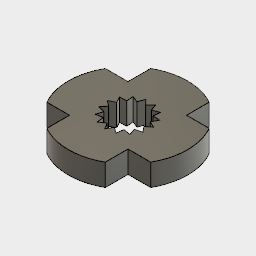
servo_horn_through_hole (Autodesk Fusion 360 design; units mm, degrees)
Autodesk Fusion 360 part; units mm, degrees
sketch "スケッチ1" plane through (0, 0, 0) normal (0, 1, 0) x (1, 0, 0)
  circle A0 centre (0, 0) radius 5.4
  line L0 (2.65, -2.65) -> (-2.65, -2.65)
  line L1 (-2.65, -2.65) -> (-2.65, 2.65)
  line L2 (-2.65, 2.65) -> (2.65, 2.65)
  line L3 (2.65, 2.65) -> (2.65, -2.65)
  line L4 (2.65, -2.65) -> (-2.65, 2.65) construction
  line L5 (-2.65, -2.65) -> (2.65, 2.65) construction
  line L6 (2.65, 2.65) -> (4.7051, 2.65)
  line L7 (2.65, 2.65) -> (2.65, 4.7051)
  line L8 (-2.65, 2.65) -> (-4.7051, 2.65)
  line L9 (-2.65, 2.65) -> (-2.65, 4.7051)
  line L10 (-2.65, -2.65) -> (-4.7051, -2.65)
  line L11 (-2.65, -2.65) -> (-2.65, -4.7051)
  line L12 (2.65, -2.65) -> (2.65, -4.7051)
  line L13 (2.65, -2.65) -> (4.7051, -2.65)
  dimension "d1" = 10.8
  dimension "d4" = 5.3
  dimension "d5" = 5.3
  constraint perpendicular L0 L1
  constraint parallel L0 L2
  constraint parallel L1 L3
  constraint horizontal L0
  constraint coincident L4
  constraint coincident L5
  constraint coincident A0
  constraint perpendicular L3 L6
  constraint perpendicular L6 L7
  constraint perpendicular L7 L8
  constraint perpendicular L8 L9
  constraint perpendicular L9 L10
  constraint perpendicular L10 L11
  constraint perpendicular L0 L12
  constraint perpendicular L12 L13
  measures "d1" diameter of A0
sketch "スケッチ2" plane through (0, 0, 0) normal (0, 1, 0) x (1, 0, 0)
  line L0 (0, -2.102) -> (0.855, -1.9203)
  line L1 (0.855, -1.9203) -> (1.5621, -1.4065)
  line L2 (1.5621, -1.4065) -> (1.9991, -0.6496)
  line L3 (1.9991, -0.6496) -> (2.0905, 0.2197)
  line L4 (2.0905, 0.2197) -> (1.8204, 1.051)
  line L5 (1.8204, 1.051) -> (1.2355, 1.7006)
  line L6 (1.2355, 1.7006) -> (0.437, 2.0561)
  line L7 (0.437, 2.0561) -> (-0.437, 2.0561)
  line L8 (-0.437, 2.0561) -> (-1.2355, 1.7006)
  line L9 (-1.2355, 1.7006) -> (-1.8204, 1.051)
  line L10 (-1.8204, 1.051) -> (-2.0905, 0.2197)
  line L11 (-2.0905, 0.2197) -> (-1.9991, -0.6496)
  line L12 (-1.9991, -0.6496) -> (-1.5621, -1.4065)
  line L13 (-1.5621, -1.4065) -> (-0.855, -1.9203)
  line L14 (-0.855, -1.9203) -> (0, -2.102)
  line L15 (0, 1.6) -> (-0.6508, 1.4617)
  line L16 (-0.6508, 1.4617) -> (-1.189, 1.0706)
  line L17 (-1.189, 1.0706) -> (-1.5217, 0.4944)
  line L18 (-1.5217, 0.4944) -> (-1.5912, -0.1672)
  line L19 (-1.5912, -0.1672) -> (-1.3856, -0.8)
  line L20 (-1.3856, -0.8) -> (-0.9405, -1.2944)
  line L21 (-0.9405, -1.2944) -> (-0.3327, -1.565)
  line L22 (-0.3327, -1.565) -> (0.3327, -1.565)
  line L23 (0.3327, -1.565) -> (0.9405, -1.2944)
  line L24 (0.9405, -1.2944) -> (1.3856, -0.8)
  line L25 (1.3856, -0.8) -> (1.5912, -0.1672)
  line L26 (1.5912, -0.1672) -> (1.5217, 0.4944)
  line L27 (1.5217, 0.4944) -> (1.189, 1.0706)
  line L28 (1.189, 1.0706) -> (0.6508, 1.4617)
  line L29 (0.6508, 1.4617) -> (0, 1.6)
  line L30 (0, -2.102) -> (0.3327, -1.565)
  line L31 (0.3327, -1.565) -> (0.855, -1.9203)
  line L32 (0.855, -1.9203) -> (0.9405, -1.2944)
  line L33 (0.9405, -1.2944) -> (1.5621, -1.4065)
  line L34 (1.5621, -1.4065) -> (1.3856, -0.8)
  line L35 (1.3856, -0.8) -> (1.9991, -0.6496)
  line L36 (1.5912, -0.1672) -> (1.9991, -0.6496)
  line L37 (1.5912, -0.1672) -> (2.0905, 0.2197)
  line L38 (2.0905, 0.2197) -> (1.5217, 0.4944)
  line L39 (1.8204, 1.051) -> (1.5217, 0.4944)
  line L40 (1.8204, 1.051) -> (1.189, 1.0706)
  line L41 (1.2355, 1.7006) -> (1.189, 1.0706)
  line L42 (1.2355, 1.7006) -> (0.6508, 1.4617)
  line L43 (0.437, 2.0561) -> (0.6508, 1.4617)
  line L44 (0.437, 2.0561) -> (0, 1.6)
  line L45 (0, 1.6) -> (-0.437, 2.0561)
  line L46 (-0.437, 2.0561) -> (-0.6508, 1.4617)
  line L47 (-1.2355, 1.7006) -> (-0.6508, 1.4617)
  line L48 (-1.2355, 1.7006) -> (-1.189, 1.0706)
  line L49 (-1.189, 1.0706) -> (-1.8204, 1.051)
  line L50 (-1.8204, 1.051) -> (-1.5217, 0.4944)
  line L51 (-1.5217, 0.4944) -> (-2.0905, 0.2197)
  line L52 (-2.0905, 0.2197) -> (-1.5912, -0.1672)
  line L53 (-1.5912, -0.1672) -> (-1.9991, -0.6496)
  line L54 (-1.9991, -0.6496) -> (-1.3856, -0.8)
  line L55 (-1.3856, -0.8) -> (-1.5621, -1.4065)
  line L56 (-1.5621, -1.4065) -> (-0.9405, -1.2944)
  line L57 (-0.855, -1.9203) -> (-0.9405, -1.2944)
  line L58 (-0.855, -1.9203) -> (-0.3327, -1.565)
  line L59 (-0.3327, -1.565) -> (0, -2.102)
extrude "押し出し1" add sketch "スケッチ1" along normal blind 2 contours A0 L3 L6 L13 | A0 L2 L7 L9 | L0 L1 L2 L3 | A0 L0 L11 L12 | A0 L1 L8 L10
extrude "押し出し2" cut sketch "スケッチ2" along normal blind 2 contours L22 L30 L59 | L23 L31 L32 | L21 L57 L58 | L15 L16 L17 L18 L19 L20 L21 L22 L23 L24 L25 L26 L27 L28 L29 | L24 L33 L34 | L20 L55 L56 | L25 L35 L36 | L19 L53 L54 | L26 L37 L38 | L18 L51 L52 | L27 L39 L40 | L17 L49 L50 | L28 L41 L42 | L16 L47 L48 | L29 L43 L44 | L15 L45 L46
